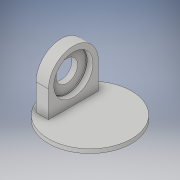
# Autodesk Inventor part: 201-
Saved by Autodesk Inventor 2018 (Build 220112000, 112)
## iProperties
Created: 2020-01-12
Part Number: 201-
Material: Generic
Document SubType Name: Modeling
Designer: Bunny320
Density: 1 g/cm^3
Appearance: Default
Author: Bunny320
Autodesk Inventor part; units mm, degrees
ref_plane "YZ Plane" through (0, 0, 0) normal (1, 0, 0) x (0, 1, 0)
ref_plane "XZ Plane" through (0, 0, 0) normal (0, 1, 0) x (-1, 0, 0)
ref_plane "XY Plane" through (0, 0, 0) normal (0, 0, 1) x (1, 0, 0)
sketch "Sketch1" plane through (0, 0, 0) normal (0, 0, 1) x (1, 0, 0)
  circle A0 centre (0, 0) radius 35
  point P0 (0, 35)
  point P1 (0, -35)
  dimension "d0" = 70
  constraints: 2 point on circle, 1 centre point, 1 coincident
  measures "d0" diameter of A0
extrude "Extrusion1" add sketch "Sketch1" along normal blind 5
sketch "Sketch3" plane through (0, 0, 5) normal (0, 0, 1) x (1, 0, 0)
  circle A0 centre (0, 0) radius 50
  dimension "d8" = 100
  constraints: 1 centre point, 1 coincident
  measures "d8" diameter of A0
extrude "Extrusion3" add sketch "Sketch3" along normal blind 5
sketch "Sketch2" plane through (0, 0, 10) normal (0, 0, 1) x (1, 0, 0)
  line L0 (-35, -30) -> (-20, -30)
  line L1 (-20, -30) -> (-20, 30)
  line L2 (-20, 30) -> (-35, 30)
  line L3 (-35, 30) -> (-35, -30)
  line L4 (-35, -30) -> (-20, 30) construction
  line L5 (-20, -30) -> (-35, 30) construction
  point P0 (0, 0)
  point P1 (-27.5, 0)
  dimension "d3" = 15
  dimension "d4" = 60
  dimension "d5" = 20
  constraints: 12 end point, 2 midpoint, 2 parallel, 1 horizontal, 1 perpendicular
  measures "d3" distance of L1.end L2.end
  measures "d4" distance of L2.end L0.start
  measures "d5" distance from line of point (0, 0) L1
extrude "Extrusion2" add sketch "Sketch2" along normal blind 62
full round fillet "Fillet1" first side at (-30, -30, 51.3333) centre faces at (-30, 10, 72) second side at (-25, 30, 51.3333)
sketch "Sketch5" plane through (0, 0, 0) normal (0, 1, 0) x (-1, 0, 0)
  line L0 (35, 215.9432) -> (32.4616, 215.9432)
  line L1 (38.0841, 42) -> (15.386, 42)
  line L2 (35, 72) -> (35, 42) projected
  line L3 (35, 55) -> (28, 55)
  line L4 (28, 55) -> (28, 65)
  line L5 (28, 65) -> (27, 65)
  line L6 (27, 65) -> (27, 65.65)
  line L7 (27, 65.65) -> (20, 65.65)
  line L8 (20, 42) -> (20, 72) projected
  point P0 (0, 0)
  dimension "d12" = 47.3
  dimension "d13" = 7
  dimension "d14" = 46
  dimension "d15" = 1
  dimension "d16" = 26
  constraints: 14 end point, 5 point on line, 4 perpendicular, 3 horizontal
  measures "d12" diameter of L7 L1
  measures "d13" distance between parallel lines of L8 L6
  measures "d14" diameter of L5 L1
  measures "d15" distance of L4.end L5.end
  measures "d16" diameter of L3 L1
revolve "Revolution1" cut sketch "Sketch5" angle 360 about axis through (-38.0841, 0, 42) along (1, 0, 0)
body "Solid1"
